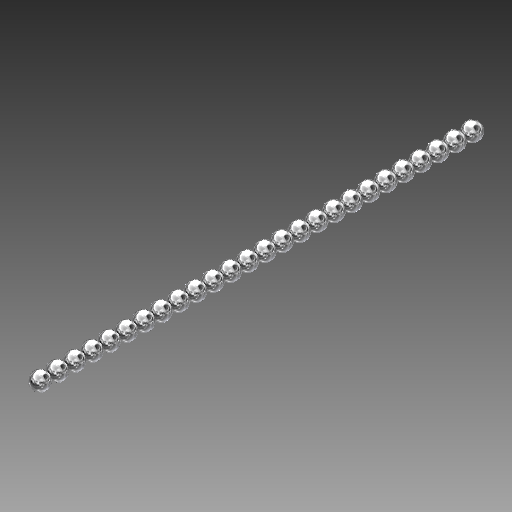
# Autodesk Inventor part: SAR330_ba
Saved by Autodesk Inventor 2019 (Build 230136000, 136)
## iProperties
Category: PARTsolutions
Company: MISUMI
Created: 2019-04-19
Part Number: SAR330_ba
Material: Aluminum 6061
Catalog Web Link: www.cadenas.de
Description: SAR3_ball-Slide Rails - Aluminum Alloy - Three - Step Slide Rails
Vendor: MISUMI
Document SubType Name: Modeling
Designer: psadmin
Manufacturer: MISUMI
Mass: 1.26179 g
Surface Area: 8.62663 cm^2
Volume: 0.467328 cm^3
Density: 2.7 g/cm^3
Appearance: Aluminum - Flat
PSOL_IDENT_0: {$CADENAS_DATA\23d-libs\misumi\metric\07_slide_rails\sar3_series\sar3_ball.prj},162 {VTYP=3D},{NB=SA
PSOL_IDENT_1: R330_ba},{LINA=SAR330},{NN=SAR3_ball},{DATE=30.03.2018 01:39:43},{GEOMDATE=01.03.2017 01:33:48},{VER
PSOL_IDENT_2: SION=},{LINEID=10},{WBVAR=NO},{WBNUMERIC=NO}  {NB=SAR330_ba},{LINA=SAR330},{KT=DUMMY},{PN=SAR330},{T
PSOL_IDENT_3: YPE=SAR3},{NO=30},{BA=25}
NN: SAR3_ball
NT: Slide Rails - Aluminum Alloy - Three - Step Slide Rails
NB: SAR330_ba
NBSYN: $PN._ba
LINA: SAR330
PN: SAR330
TYPE: SAR3
NO: 30
SUPPLIER: MISUMI
ARTICLENO: SAR330_ba
BOMINFO: SAR330
CREATOR: CADENAS GmbH
Title: SAR330
Author: Cadenas PARTsolutions
Comments: Slide Rails - Aluminum Alloy - Three - Step Slide Rails
Autodesk Inventor part; units mm, degrees
sketch "Sketch_1" plane through (0, 0, 0) normal (1, 0, 0) x (0, 1, 0)
  line L0 (0, 0) -> (0, 81.25)
  line L1 (0, 81.25) -> (0.025, 81.25)
  line L2 (0.025, 81.25) -> (0.025, 0)
  line L3 (0.025, 0) -> (0, 0)
  line L4 (0, 0) -> (0, 81.25)
  constraints: 10 end point
revolve "Revolution1" add sketch "Sketch_1" angle 360 about axis through (0, 0, 0) along (0, 0, -1)
sketch "Sketch_2" plane through (0, 0, 0) normal (1, 0, 0) x (0, 1, 0)
  line L0 (0, -50) -> (0, 50)
  arc A0 (0, -1.625) -> (0, 1.625) centre (0, 0) ccw
  line L1 (0, -1.625) -> (0, 1.625)
  constraints: 4 end point, 2 point on circle, 1 centre point
revolve "Revolution2" add sketch "Sketch_2" angle 360 about axis through (0, 0, -50) along (0, 0, -1)
pattern_linear "Rectangular Pattern1" count 26 spacing 3.25 along (0, 0, 1) of "Revolution2"
ref_plane "to_body_XY" through (0, 0, 0) normal (0, 0, -1) x (1, 0, 0)
ref_plane "to_body_YZ" through (0, 0, 0) normal (1, 0, 0) x (0, -1, 0)
ref_plane "to_body_ZX" through (0, 0, 0) normal (0, -1, 0) x (0, 0, -1)
body "Solid1"
